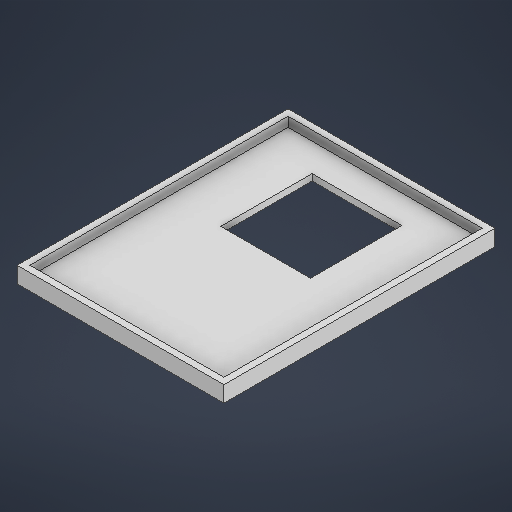
# Autodesk Inventor part: Tampa
Saved by Autodesk Inventor 2025 (Build 290162010, 162A)
## iProperties
Created: 2024-08-10
Part Number: Tampa
Material: Generic
Document SubType Name: Modeling
Designer: GabrielDBN
Density: 1 g/cm^3
Appearance: Default
Author: GabrielDBN
Autodesk Inventor part; units mm, degrees
ref_plane "YZ Plane" through (0, 0, 0) normal (1, 0, 0) x (0, 1, 0)
ref_plane "XZ Plane" through (0, 0, 0) normal (0, 1, 0) x (-1, 0, 0)
ref_plane "XY Plane" through (0, 0, 0) normal (0, 0, 1) x (1, 0, 0)
sketch "Sketch1" plane through (0, 0, 0) normal (0, 1, 0) x (-1, 0, 0)
  line L0 (30.9809, 37.6192) -> (-29.5191, 37.6192)
  line L1 (30.9809, 37.6192) -> (30.9809, -42.8808)
  line L2 (30.9809, -42.8808) -> (-29.5191, -42.8808)
  line L3 (-29.5191, -42.8808) -> (-29.5191, 37.6192)
  line L4 (32.9809, 39.6192) -> (-31.5191, 39.6192)
  line L5 (-31.5191, 39.6192) -> (-31.5191, -44.8808)
  line L6 (-31.5191, -44.8808) -> (32.9809, -44.8808)
  line L7 (32.9809, -44.8808) -> (32.9809, 39.6192)
  line L8 (14.7309, -34.1308) -> (14.7309, -5.6308)
  line L9 (14.7309, -5.6308) -> (-13.2691, -5.6308)
  line L10 (-13.2691, -5.6308) -> (-13.2691, -34.1308)
  line L11 (14.7309, -34.1308) -> (-13.2691, -34.1308)
  point P0 (0, 0)
  dimension "d0" = 60.5
  dimension "d1" = 80.5
  dimension "d6" = 64.5
  dimension "d7" = 84.5
  dimension "d11" = 28.5
  dimension "d17" = 28
  constraints: 24 end point, 4 horizontal, 4 perpendicular, 2 vertical
  measures "d0" distance of L0.start L0.end
  measures "d1" distance of L0.start L1.end
  measures "d6" distance of L4.start L4.end
  measures "d7" distance of L6.end L4.start
  measures "d11" distance of L8.start L8.end
  measures "d17" distance of L8.end L9.end
extrude "Extrusion1" add sketch "Sketch1" along normal blind 2 contours L1 L2 L3 L0
extrude "Extrusion2" add sketch "Sketch1" along normal blind 5 contours L7 L6 L5 L4
body "Solid1"
